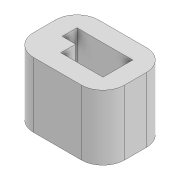
# Autodesk Inventor part: Plugholder
Saved by Autodesk Inventor 2021 (Build 250183000, 183)
## iProperties
Created: 2021-08-21
Part Number: Plugholder
Material: Generisch
Document SubType Name: Modeling
Designer: Rama
Density: 1 g/cm^3
Appearance: Vorgabe
Author: Rama
Autodesk Inventor part; units mm, degrees
ref_plane "YZ Plane" through (0, 0, 0) normal (1, 0, 0) x (0, 1, 0)
ref_plane "XZ Plane" through (0, 0, 0) normal (0, 1, 0) x (-1, 0, 0)
ref_plane "XY Plane" through (0, 0, 0) normal (0, 0, 1) x (1, 0, 0)
sketch "Skizze1" plane through (0, 0, 0) normal (0, 1, 0) x (-1, 0, 0)
  line L0 (-5.15, 2.75) -> (2.65, 2.75)
  line L1 (2.65, 2.75) -> (2.65, 0)
  line L2 (2.65, 0) -> (5.15, 0)
  line L3 (5.15, 0) -> (5.15, -2.75)
  line L4 (5.15, -2.75) -> (-5.15, -2.75)
  line L5 (-5.15, -2.75) -> (-5.15, 2.75)
  line L6 (8.4, 6) -> (-8.4, 6)
  line L7 (-8.4, 6) -> (-8.4, -6)
  line L8 (-8.4, -6) -> (8.4, -6)
  line L9 (8.4, -6) -> (8.4, 6)
  line L10 (8.4, 6) -> (-8.4, -6) construction
  line L11 (-8.4, 6) -> (8.4, -6) construction
  point P0 (0, 0)
  point P1 (0, 0)
  dimension "d0" = 16.8
  dimension "d1" = 12
  dimension "d2" = 5.5
  dimension "d3" = 10.3
  dimension "d4" = 2.75
  dimension "d5" = 7.8
  dimension "d6" = 2.75
  dimension "d7" = 3.25
  dimension "d8" = 3.25
  constraints: 24 end point, 2 midpoint, 2 parallel, 1 coincident, 1 horizontal, 1 perpendicular
  measures "d0" distance of L8.end L7.end
  measures "d1" distance of L7.end L6.end
  measures "d2" distance between parallel lines of L4 L0
  measures "d3" distance between parallel lines of L3 L5
  measures "d4" distance of L0.end L1.end
  measures "d5" distance between parallel lines of L5 L1
  measures "d6" distance between parallel lines of L4 L2
  measures "d7" distance between parallel lines of L0 L6
  measures "d8" distance between parallel lines of L8 L4
extrude "Extrusion1" add sketch "Skizze1" along normal blind 12
fillet "Rundung1" radius 4 4 edges at (8.4, 6, -6) (8.4, 6, 6) (-8.4, 6, -6) (-8.4, 6, 6)
sketch "Skizze3" plane through (4.4, 0, -6) normal (0, 0, -1) x (-1, 0, 0)
  line L0 (8.075, 6) -> (6.525, 6)
  line L1 (6.525, 6) -> (4.3724, 2.7478)
  line L2 (8.075, 6) -> (5.9224, 2.7478)
  line L3 (8.075, 6) -> (11.975, 6) construction
  line L4 (5.9224, 2.7478) -> (4.3724, 2.7478)
  line L5 (3.0224, 2.7478) -> (7.3276, 9.2522)
  line L6 (3.0224, 2.7478) -> (10.8224, 2.7478) construction
  line L7 (7.3276, 9.2522) -> (5.7776, 9.2522)
  line L8 (7.3276, 9.2522) -> (8.8776, 9.2522) construction
  line L9 (5.7776, 9.2522) -> (1.4724, 2.7478)
  line L10 (1.4724, 2.7478) -> (3.0224, 2.7478)
  line L11 (4.4276, 9.2522) -> (2.8776, 9.2522)
  line L12 (2.8776, 9.2522) -> (0.725, 6)
  line L13 (0.725, 6) -> (2.275, 6)
  line L14 (0.725, 6) -> (2.275, 6) construction
  line L15 (2.275, 6) -> (4.4276, 9.2522)
  line L16 (-4, 12) -> (-4, 0) projected
  line L17 (12.8, 0) -> (12.8, 12) projected
  line L18 (0, 12) -> (8.8, 12) projected
  line L19 (0, 0) -> (8.8, 0) projected
  point P0 (4.4, 0)
  point P1 (0, 12.9522)
  dimension "d21" = 3.9
  dimension "d22" = 123.5
  dimension "d23" = 3.9
  dimension "d24" = 123.5
  dimension "d25" = 7.8
  dimension "d26" = 56.5
  dimension "d27" = 1.55
  dimension "d28" = 1.55
  dimension "d29" = 1.55
  dimension "d30" = 180
  dimension "d31" = 123.5
  dimension "d32" = 1.55
  dimension "d33" = 3.9
  dimension "d34" = 123.5
  dimension "d35" = 1.55
  dimension "d36" = 0
  dimension "d37" = 1.35
  dimension "d38" = 1.35
  dimension "d39" = 7.35
  dimension "d42" = 3.7
  dimension "d43" = 0
  dimension "d50" = 4.725
  dimension "d51" = 4.725
  dimension "d52" = 2.7479
  dimension "d53" = 2.7479
  constraints: 32 end point, 8 horizontal, 4 equal length, 3 parallel, 1 point on line
  measures "d21" distance of L0.end L1.end
  measures "d22" angle of L1 L0
  measures "d23" distance of L0.start L2.end
  measures "d24" angle of L2 L3
  measures "d25" distance of L5.start L5.end
  measures "d26" angle of L6 L5
  measures "d27" distance of L0.start L0.end
  measures "d28" distance of L2.end L1.end
  measures "d29" distance of L5.end L7.end
  measures "d30" angle of L7 L8
  measures "d31" angle of L9 L7
  measures "d32" distance of L11.start L11.end
  measures "d33" distance of L11.end L12.end
  measures "d34" angle of L12 L11
  measures "d35" distance of L12.end L13.end
  measures "d36" distance between parallel lines of L13 L14
  measures "d37" distance of L5.start L1.end
  measures "d38" distance of L11.start L7.end
  measures "d39" distance of L12.end L0.start
  measures "d42" distance from line of point (0, 12.952) L11
  measures "d43" distance between parallel lines of L7 L11
  measures "d50" distance from line of L12.end L16
  measures "d51" distance from line of L17 L0.start
  measures "d52" distance between parallel lines of L18 L11
  measures "d53" distance between parallel lines of L19 L10
extrude "Extrusion3" cut sketch "Skizze3" against normal blind 0.5
chamfer "Fase2" distance 0.5 angle 45 6 edges at (-2.1526, 9.2522, -5.5) (-2.9, 6, -5.5) (0.7474, 9.2522, -5.5) (2.9, 6, -5.5) (2.1526, 2.7478, -5.5) (-0.7474, 2.7478, -5.5)
equation "\"d0\" = d3 + 2 * d7"
equation "\"d7\" = d8"
equation "\"d37\" = d38"
equation "\"d50\" = d51"
equation "\"d52\" = d53"
